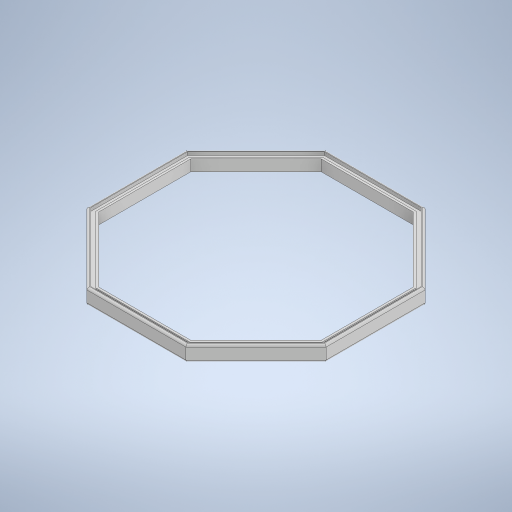
# Autodesk Inventor part: OV-PAM_ring_2
Saved by Autodesk Inventor 2024 (Build 280153000, 153)
## iProperties
Created: 2023-06-19
Part Number: OV-PAM_ring_2
Material: 일반
Document SubType Name: Modeling
Designer: jsw
Density: 1 g/cm^3
Appearance: 기본값
Author: jsw
Autodesk Inventor part; units mm, degrees
ref_plane "YZ Plane" through (0, 0, 0) normal (1, 0, 0) x (0, 1, 0)
ref_plane "XZ Plane" through (0, 0, 0) normal (0, 1, 0) x (-1, 0, 0)
ref_plane "XY Plane" through (0, 0, 0) normal (0, 0, 1) x (1, 0, 0)
sketch "스케치1" plane through (0, 0, 0) normal (0, 1, 0) x (-1, 0, 0)
  line L0 (-65.1838, 27) -> (-27, 65.1838)
  line L1 (-27, 65.1838) -> (27, 65.1838)
  line L2 (27, 65.1838) -> (65.1838, 27)
  line L3 (65.1838, 27) -> (65.1838, -27)
  line L4 (65.1838, -27) -> (27, -65.1838)
  line L5 (27, -65.1838) -> (-27, -65.1838)
  line L6 (-27, -65.1838) -> (-65.1838, -27)
  line L7 (-65.1838, -27) -> (-65.1838, 27)
  line L8 (68.3838, 28.3255) -> (68.3838, -28.3255)
  line L9 (68.3838, -28.3255) -> (28.3255, -68.3838)
  line L10 (28.3255, -68.3838) -> (-28.3255, -68.3838)
  line L11 (-28.3255, -68.3838) -> (-68.3838, -28.3255)
  line L12 (-68.3838, -28.3255) -> (-68.3838, 28.3255)
  line L13 (-68.3838, 28.3255) -> (-28.3255, 68.3838)
  line L14 (-28.3255, 68.3838) -> (28.3255, 68.3838)
  line L15 (28.3255, 68.3838) -> (68.3838, 28.3255)
  point P0 (0, 0)
  point P1 (0, 0)
  point P2 (0, 0)
  dimension "d0" = 54
  dimension "d1" = 3.2
  constraints: 32 end point, 2 coincident, 2 horizontal, 34 other
  measures "d0" distance of L2.end L3.end
  measures "d1" distance between parallel lines of L8 L3
extrude "돌출1" add sketch "스케치1" along normal blind 8.8 contours L0 L1 L2 L3 L4 L5 L6 L7 | L8 L9 L10 L11 L12 L13 L14 L15
sketch "스케치3" plane through (0, 0, 0) normal (0, -1, 0) x (1, 0, 0)
  line L0 (-26.8343, 64.7838) -> (26.8343, 64.7838)
  line L1 (26.8343, 64.7838) -> (64.7838, 26.8343)
  line L2 (64.7838, 26.8343) -> (64.7838, -26.8343)
  line L3 (64.7838, -26.8343) -> (26.8343, -64.7838)
  line L4 (26.8343, -64.7838) -> (-26.8343, -64.7838)
  line L5 (-26.8343, -64.7838) -> (-64.7838, -26.8343)
  line L6 (-64.7838, -26.8343) -> (-64.7838, 26.8343)
  line L7 (-64.7838, 26.8343) -> (-26.8343, 64.7838)
  line L8 (-27.6627, 66.7838) -> (27.6627, 66.7838)
  line L9 (27.6627, 66.7838) -> (66.7838, 27.6627)
  line L10 (66.7838, 27.6627) -> (66.7838, -27.6627)
  line L11 (66.7838, -27.6627) -> (27.6627, -66.7838)
  line L12 (27.6627, -66.7838) -> (-27.6627, -66.7838)
  line L13 (-27.6627, -66.7838) -> (-66.7838, -27.6627)
  line L14 (-66.7838, -27.6627) -> (-66.7838, 27.6627)
  line L15 (-66.7838, 27.6627) -> (-27.6627, 66.7838)
  line L16 (-28.3255, 68.3838) -> (28.3255, 68.3838) projected
  point P0 (0, 0)
  point P1 (0, 0)
  point P2 (0, 0)
  point P3 (0, 0)
  dimension "d9" = 2
  dimension "d144" = 1.6
  constraints: 32 end point, 3 coincident, 2 horizontal, 34 other
  measures "d9" distance between parallel lines of L8 L0
  measures "d144" distance between parallel lines of L8 L16
extrude "돌출3" cut sketch "스케치3" against normal blind 1.8
sketch "스케치14" plane through (0, 0, 0) normal (0, -1, 0) x (1, 0, 0)
  line L0 (64.7838, 26.8343) -> (26.8343, 64.7838) projected
  line L1 (26.8343, 64.7838) -> (-26.8343, 64.7838) projected
  line L2 (-26.8343, 64.7838) -> (-64.7838, 26.8343) projected
  line L3 (-64.7838, 26.8343) -> (-64.7838, -26.8343) projected
  line L4 (-64.7838, -26.8343) -> (-26.8343, -64.7838) projected
  line L5 (-26.8343, -64.7838) -> (26.8343, -64.7838) projected
  line L6 (26.8343, -64.7838) -> (64.7838, -26.8343) projected
  line L7 (64.7838, -26.8343) -> (64.7838, 26.8343) projected
  point P0 (0, 0)
extrude "돌출16" cut sketch "스케치14" against normal blind 1.2
sketch "스케치15" plane through (0, 1.2, 0) normal (0, -1, 0) x (1, 0, 0)
  line L0 (-26.3373, 63.5838) -> (26.3373, 63.5838)
  line L1 (26.3373, 63.5838) -> (63.5838, 26.3373)
  line L2 (63.5838, 26.3373) -> (63.5838, -26.3373)
  line L3 (63.5838, -26.3373) -> (26.3373, -63.5838)
  line L4 (26.3373, -63.5838) -> (-26.3373, -63.5838)
  line L5 (-26.3373, -63.5838) -> (-63.5838, -26.3373)
  line L6 (-63.5838, -26.3373) -> (-63.5838, 26.3373)
  line L7 (-63.5838, 26.3373) -> (-26.3373, 63.5838)
  line L8 (-26.8343, 64.7838) -> (26.8343, 64.7838) projected
  point P0 (0, 0)
  point P1 (0, 0)
  dimension "d140" = 1.2
  constraints: 16 end point, 1 coincident, 1 horizontal, 17 other
  measures "d140" distance between parallel lines of L0 L8
extrude "돌출17" cut sketch "스케치15" against normal up to surface (7.6 mm away)
ref_plane "작업 평면3" through (0, 4.4, 0) normal (0, -1, 0) x (1, 0, 0)
mirror "미러6" about plane through (0, 4.4, 0) normal (0, -1, 0) of "돌출3", "돌출16"
fillet "모깎기2" radius 1.2 16 edges at (0, 0, 68.3838) (-48.3546, 0, 48.3546) (-68.3838, 0, 0) (-48.3546, 0, -48.3546) (0, 0, -68.3838) (48.3546, 0, -48.3546) (68.3838, 0, 0) (48.3546, 0, 48.3546) (-48.3546, 8.8, 48.3546) (-68.3838, 8.8, 0) (-48.3546, 8.8, -48.3546) (0, 8.8, -68.3838) (48.3546, 8.8, -48.3546) (68.3838, 8.8, 0) (48.3546, 8.8, 48.3546) (0, 8.8, 68.3838)
